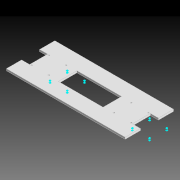
# Autodesk Inventor part: KB33-046-004-019 - Площадка под драйверы
Saved by Autodesk Inventor 2020 (Build 240168000, 168)
## iProperties
Created: 2021-08-02
Part Number: KB33-046-004-019 - Площадка под драйверы
Material: Типовые
Document SubType Name: Modeling
Designer: Петров Иван
Density: 1 g/cm^3
Appearance: По умолчанию
Mass: 84.9896 g
Surface Area: 472.363 cm^2
Volume: 84.9896 cm^3
Author: Петров Иван
Autodesk Inventor part; units mm, degrees
ref_plane "YZ Plane" through (0, 0, 0) normal (1, 0, 0) x (0, 1, 0)
ref_plane "XZ Plane" through (0, 0, 0) normal (0, 1, 0) x (-1, 0, 0)
ref_plane "XY Plane" through (0, 0, 0) normal (0, 0, 1) x (1, 0, 0)
sketch "Эскиз1" plane through (0, 0, 0) normal (0, 1, 0) x (-1, 0, 0)
  line L0 (-127.5, 51.9915) -> (127.5, 51.9915)
  line L1 (127.5, 51.9915) -> (127.5, -51.9915)
  line L2 (127.5, -51.9915) -> (-127.5, -51.9915)
  line L3 (-127.5, -51.9915) -> (-127.5, 51.9915)
  line L4 (-48, 20) -> (48, 20)
  line L5 (48, 20) -> (48, -20)
  line L6 (48, -20) -> (-48, -20)
  line L7 (-48, -20) -> (-48, 20)
  line L8 (-48, 20) -> (48, -20) construction
  line L9 (48, 20) -> (-48, -20) construction
  line L10 (127.5, 19.4125) -> (110.25, 19.4125)
  line L11 (110.25, 19.4125) -> (110.25, -19.4125)
  line L12 (110.25, -19.4125) -> (127.5, -19.4125)
  line L13 (127.5, -19.4125) -> (127.5, 19.4125)
  line L14 (48, 0) -> (57.4345, 0)
  line L15 (0, 0) -> (0, -38.2708)
  line L16 (-127.5, 19.4125) -> (-110.25, 19.4125)
  line L17 (-110.25, 19.4125) -> (-110.25, -19.4125)
  line L18 (-110.25, -19.4125) -> (-127.5, -19.4125)
  line L19 (-127.5, -19.4125) -> (-127.5, 19.4125)
  dimension "d0" = 103.983
  dimension "d1" = 255
  dimension "d2" = 96
  dimension "d3" = 40
  dimension "d4" = 38.825
  dimension "d5" = 17.25
  constraints: 40 end point, 6 parallel, 4 horizontal, 4 symmetric about line, 3 midpoint, 3 perpendicular, 1 point on line, 1 vertical, 2 other
  measures "d0" distance of L0.end L1.end
  measures "d1" distance of L1.end L2.end
  measures "d2" distance of L5.end L6.end
  measures "d3" distance of L4.end L5.end
  measures "d4" distance of L10.end L11.end
  measures "d5" distance between parallel lines of L11 L1
extrude "Выдавливание1" add sketch "Эскиз1" along normal blind 4 contours L0 L1 L10 L11 L12 L2 L3 L18 L17 L16
sketch "Эскиз2" plane through (0, 0, 0) normal (0, -1, 0) x (1, 0, 0)
  circle A0 centre (40, 36) radius 1.85 projected
  circle A1 centre (40, -36) radius 1.85 projected
  circle A2 centre (-40, -36) radius 1.85 projected
  circle A3 centre (-40, 36) radius 1.85 projected
  point P0 (0, 0)
extrude "Выдавливание2" cut sketch "Эскиз2" against normal blind 3
sketch "Эскиз3" plane through (0, 0, 0) normal (0, -1, 0) x (1, 0, 0)
  circle A0 centre (-106.875, 18.5) radius 1.5 projected
  circle A1 centre (-69.875, 18.5) radius 1.5 projected
  circle A2 centre (-106.875, -18.5) radius 1.5 projected
  circle A3 centre (-69.875, -18.5) radius 1.5 projected
  circle A4 centre (69.875, -18.5) radius 1.5 projected
  circle A5 centre (69.875, 18.5) radius 1.5 projected
  circle A6 centre (106.875, 18.5) radius 1.5 projected
  circle A7 centre (106.875, -18.5) radius 1.5 projected
  point P0 (0, 0)
extrude "Выдавливание3" cut sketch "Эскиз3" against normal blind 4
